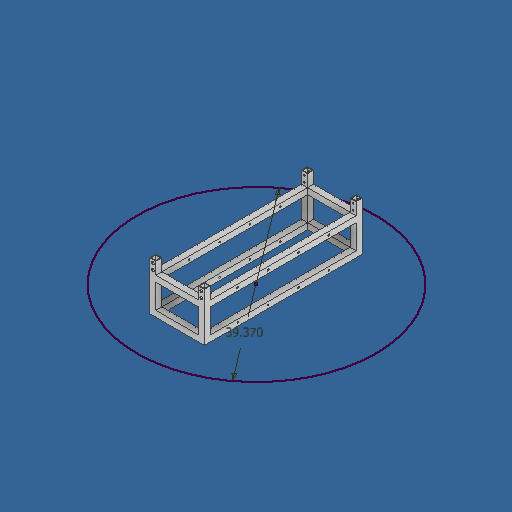
# Autodesk Inventor part: Placeholder_ChassisMain
Saved by Autodesk Inventor 2023 (Build 270158030, 158C)
## iProperties
Created: 2022-10-13
Part Number: Placeholder_ChassisMain
Material: Air
Document SubType Name: Modeling
Designer: kumpu
Density: 0.0012 g/cm^3
Appearance: Aluminum - Dark
Mass: 1.33214 g
Surface Area: 7008.81 cm^2
Volume: 1110.12 cm^3
Author: kumpu
Autodesk Inventor part; units mm, degrees
ref_plane "YZ Plane" through (0, 0, 0) normal (1, 0, 0) x (0, 1, 0)
ref_plane "XZ Plane" through (0, 0, 0) normal (0, 1, 0) x (-1, 0, 0)
ref_plane "XY Plane" through (0, 0, 0) normal (0, 0, 1) x (1, 0, 0)
sketch "Sketch1" plane through (0, 0, 0) normal (0, 1, 0) x (-1, 0, 0)
  line L0 (114.3, 330.2) -> (88.9, 330.2)
  line L1 (88.9, 330.2) -> (88.9, 304.8)
  line L2 (88.9, 304.8) -> (114.3, 304.8)
  line L3 (114.3, 304.8) -> (114.3, 330.2)
  line L4 (114.3, 330.2) -> (88.9, 304.8) construction
  line L5 (88.9, 330.2) -> (114.3, 304.8) construction
  line L6 (111.125, 327.025) -> (92.075, 327.025)
  line L7 (92.075, 327.025) -> (92.075, 307.975)
  line L8 (92.075, 307.975) -> (111.125, 307.975)
  line L9 (111.125, 307.975) -> (111.125, 327.025)
  line L10 (111.125, 327.025) -> (92.075, 307.975) construction
  line L11 (92.075, 327.025) -> (111.125, 307.975) construction
  point P0 (0, 0)
  point P1 (101.6, 317.5)
  point P2 (101.6, 317.5)
  dimension "d0" = 25.4
  dimension "d1" = 3.175
  dimension "d2" = 304.8
  dimension "d3" = 88.9
  constraints: 24 end point, 5 midpoint, 4 parallel, 3 perpendicular, 2 horizontal, 1 point on line
  measures "d0" distance of L2.end L0.start
  measures "d1" distance between parallel lines of L2 L8
  measures "d2" distance from line of point (0, 0) L2
  measures "d3" distance from line of point (0, 0) L1
extrude "Extrusion1" add sketch "Sketch1" along normal blind 177.8 and the other way blind 25.4
sketch "Sketch2" plane through (-88.9, -25.4, 304.8) normal (1, 0, 0) x (0, 0, -1)
  line L0 (-25.4, 25.4) -> (0, 25.4)
  line L1 (0, 25.4) -> (0, 0)
  line L2 (0, 0) -> (-25.4, 0)
  line L3 (-25.4, 0) -> (-25.4, 25.4)
  line L4 (-25.4, 25.4) -> (0, 0) construction
  line L5 (0, 25.4) -> (-25.4, 0) construction
  line L6 (-22.225, 22.225) -> (-3.175, 22.225)
  line L7 (-3.175, 22.225) -> (-3.175, 3.175)
  line L8 (-3.175, 3.175) -> (-22.225, 3.175)
  line L9 (-22.225, 3.175) -> (-22.225, 22.225)
  line L10 (-22.225, 22.225) -> (-3.175, 3.175) construction
  line L11 (-3.175, 22.225) -> (-22.225, 3.175) construction
  line L12 (-25.4, 152.4) -> (0, 152.4)
  line L13 (0, 152.4) -> (0, 127)
  line L14 (0, 127) -> (-25.4, 127)
  line L15 (-25.4, 127) -> (-25.4, 152.4)
  line L16 (-25.4, 152.4) -> (0, 127) construction
  line L17 (0, 152.4) -> (-25.4, 127) construction
  line L18 (-22.225, 149.225) -> (-3.175, 149.225)
  line L19 (-3.175, 149.225) -> (-3.175, 130.175)
  line L20 (-3.175, 130.175) -> (-22.225, 130.175)
  line L21 (-22.225, 130.175) -> (-22.225, 149.225)
  line L22 (-22.225, 149.225) -> (-3.175, 130.175) construction
  line L23 (-3.175, 149.225) -> (-22.225, 130.175) construction
  point P0 (304.8, 25.4)
  point P1 (-12.7, 12.7)
  point P2 (-12.7, 12.7)
  point P3 (-12.7, 139.7)
  dimension "d8" = 25.4
  dimension "d9" = 3.175
  dimension "d10" = 101.6
  constraints: 48 end point, 9 midpoint, 8 parallel, 4 equal length, 4 horizontal, 4 perpendicular, 4 point on line, 1 collinear
  measures "d8" distance of L12.end L13.end
  measures "d9" distance between parallel lines of L1 L7
  measures "d10" distance between parallel lines of L0 L14
extrude "Extrusion2" add sketch "Sketch2" along normal blind 88.9
sketch "Sketch3" plane through (-88.9, 177.8, 304.8) normal (0, 0, -1) x (-1, 0, 0)
  line L0 (0, -50.8) -> (25.4, -50.8)
  line L1 (25.4, -50.8) -> (25.4, -76.2)
  line L2 (25.4, -76.2) -> (0, -76.2)
  line L3 (0, -76.2) -> (0, -50.8)
  line L4 (0, -50.8) -> (25.4, -76.2) construction
  line L5 (25.4, -50.8) -> (0, -76.2) construction
  line L6 (3.175, -53.975) -> (22.225, -53.975)
  line L7 (22.225, -53.975) -> (22.225, -73.025)
  line L8 (22.225, -73.025) -> (3.175, -73.025)
  line L9 (3.175, -73.025) -> (3.175, -53.975)
  line L10 (3.175, -53.975) -> (22.225, -73.025) construction
  line L11 (22.225, -53.975) -> (3.175, -73.025) construction
  line L12 (0, -177.8) -> (25.4, -177.8)
  line L13 (25.4, -177.8) -> (25.4, -203.2)
  line L14 (25.4, -203.2) -> (0, -203.2)
  line L15 (0, -203.2) -> (0, -177.8)
  line L16 (0, -177.8) -> (25.4, -203.2) construction
  line L17 (25.4, -177.8) -> (0, -203.2) construction
  line L18 (3.175, -180.975) -> (22.225, -180.975)
  line L19 (22.225, -180.975) -> (22.225, -200.025)
  line L20 (22.225, -200.025) -> (3.175, -200.025)
  line L21 (3.175, -200.025) -> (3.175, -180.975)
  line L22 (3.175, -180.975) -> (22.225, -200.025) construction
  line L23 (22.225, -180.975) -> (3.175, -200.025) construction
  point P0 (-88.9, -177.8)
  point P1 (12.7, -63.5)
  point P2 (12.7, -63.5)
  point P3 (12.7, -190.5)
  point P4 (12.7, -190.5)
  point P5 (22.225, -63.5)
  point P6 (25.4, -203.2)
  dimension "d13" = 25.4
  dimension "d14" = 3.175
  constraints: 48 end point, 11 midpoint, 8 parallel, 7 point on line, 4 horizontal, 4 perpendicular, 3 equal length
  measures "d13" distance of L0.end L1.end
  measures "d14" distance from line of L1 point (22.225, -63.5)
extrude "Extrusion3" add sketch "Sketch3" along normal blind 304.8
sketch "Sketch4" plane through (-114.3, 177.8, 330.2) normal (0, 0, 1) x (1, 0, 0)
  line L0 (0, 0) -> (25.4, 0) projected
  line L1 (25.4, 0) -> (25.4, -50.8) projected
  point P0 (114.3, -177.8)
  point P1 (12.7, -12.7)
  dimension "d17" = 12.7
  dimension "d18" = 12.7
  measures "d17" distance from line of L0 point (12.7, -12.7)
  measures "d18" distance from line of L1 point (12.7, -12.7)
hole "Hole1" at (-101.6, 165.1, 330.2) direction (0, 0, -1) diameter 6.35 end through all
sketch "Sketch5" plane through (-114.3, 177.8, 330.2) normal (0, 0, 1) x (1, 0, 0)
  line L0 (25.4, 0) -> (25.4, -50.8) projected
  line L1 (0, 0) -> (25.4, 0) projected
  point P0 (114.3, -177.8)
  point P1 (12.7, -38.1)
  dimension "d26" = 12.7
  dimension "d27" = 38.1
  measures "d26" distance from line of L0 point (12.7, -38.1)
  measures "d27" distance from line of L1 point (12.7, -38.1)
hole "Hole2" at (-101.6, 139.7, 330.2) direction (0, 0, -1) diameter 6.35 end through all
sketch "Sketch6" plane through (-114.3, 177.8, 330.2) normal (0, 0, 1) x (1, 0, 0)
  circle A0 centre (12.7, -38.1) radius 3.175 projected
  point P0 (114.3, -177.8)
  constraints: 1 coincident
hole "Hole3" at (-101.6, 139.7, 330.2) direction (0, 0, -1) diameter 12.7 depth 12.7 tip angle 118
sketch "Sketch7" plane through (-114.3, 177.8, 330.2) normal (0, 0, 1) x (1, 0, 0)
  circle A0 centre (12.7, -12.7) radius 3.175 projected
  point P0 (114.3, -177.8)
  constraints: 1 coincident
hole "Hole4" at (-101.6, 165.1, 330.2) direction (0, 0, -1) diameter 12.7 depth 12.7 tip angle 118
mirror "Mirror1" about plane through (0, 0, 0) normal (1, 0, 0)
mirror "Mirror2" about plane through (0, 0, 0) normal (0, 0, 1)
sketch "Sketch8" plane through (0, -25.4, 0) normal (0, -1, 0) x (1, 0, 0)
  circle A0 centre (0, 0) radius 500
  dimension "d49" = 1000
  constraints: 1 centre point, 1 coincident
  measures "d49" diameter of A0
sketch "Sketch9" plane through (114.3, -25.4, 330.2) normal (1, 0, 0) x (0, 0, -1)
  line L0 (0, 0) -> (0, 203.2) projected
  line L1 (0, 0) -> (660.4, 0) projected
  point P0 (330.2, 25.4)
  point P1 (139.7, 12.7)
  dimension "d50" = 139.7
  dimension "d51" = 12.7
  measures "d50" distance from line of L0 point (139.7, 12.7)
  measures "d51" distance from line of L1 point (139.7, 12.7)
hole "Hole5" at (114.3, -12.7, 190.5) direction (-1, 0, 0) diameter 7.1374 end through all clearance for "Flat Head Machine Screw (82)" size "1/4" standard "Ansi Unified Screw Threads"
sketch "Sketch10" plane through (114.3, -25.4, 330.2) normal (1, 0, 0) x (0, 0, -1)
  line L0 (25.4, 152.4) -> (635, 152.4) projected
  line L1 (0, 0) -> (0, 203.2) projected
  point P0 (330.2, 25.4)
  point P1 (139.7, 139.7)
  dimension "d59" = 12.7
  dimension "d60" = 139.7
  measures "d59" distance from line of L0 point (139.7, 139.7)
  measures "d60" distance from line of L1 point (139.7, 139.7)
hole "Hole6" at (114.3, 114.3, 190.5) direction (-1, 0, 0) diameter 6.7564 end through all counterbore diameter 7.9502 counterbore depth 4.7752 clearance for "Hex Head Bolt" size "1/4" standard "Ansi Unified Screw Threads"
sketch "Sketch11" plane through (-114.3, -25.4, 330.2) normal (-1, 0, 0) x (0, 0, 1)
  circle A0 centre (-139.7, 139.7) radius 3.3782 projected
  point P0 (-330.2, 25.4)
  constraints: 1 coincident
hole "Hole7" at (-114.3, 114.3, 190.5) direction (1, 0, 0) diameter 6.7564 end through all counterbore diameter 8.382 counterbore depth 4.7752
pattern_linear "Rectangular Pattern1" count 4 spacing 127 along (0, 0, -1) of "Hole5", "Hole6", "Hole7"
body "Solid1"
